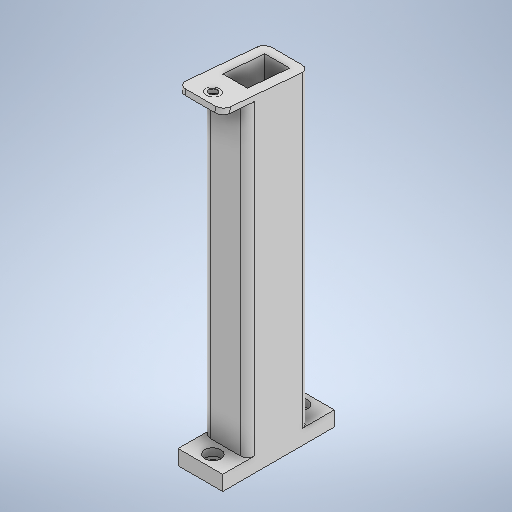
# Autodesk Inventor part: Path Holder
Saved by Autodesk Inventor 2025.4 (Build 294407000, 407)
## iProperties
Created: 2026-04-06
Part Number: Path Holder
Material: Generic
Document SubType Name: Modeling
Designer: lenovo
Density: 1 g/cm^3
Appearance: Default
Author: lenovo
Autodesk Inventor part; units mm, degrees
ref_plane "YZ Plane" through (0, 0, 0) normal (1, 0, 0) x (0, 1, 0)
ref_plane "XZ Plane" through (0, 0, 0) normal (0, 1, 0) x (-1, 0, 0)
ref_plane "XY Plane" through (0, 0, 0) normal (0, 0, 1) x (1, 0, 0)
sketch "Sketch2" plane through (0, 0, 0) normal (0, 1, 0) x (-1, 0, 0)
  line L0 (5, 8.5) -> (-5, 8.5)
  line L1 (-5, 8.5) -> (-5, -8.5)
  line L2 (-5, -8.5) -> (5, -8.5)
  line L3 (5, -8.5) -> (5, 8.5)
  line L4 (5, 8.5) -> (-5, -8.5) construction
  line L5 (-5, 8.5) -> (5, -8.5) construction
  line L6 (9, 12.5) -> (-9, 12.5)
  line L7 (-9, 12.5) -> (-9, -12.5)
  line L8 (-9, -12.5) -> (9, -12.5)
  line L9 (9, -12.5) -> (9, 12.5)
  point P0 (0, 0)
  dimension "d0" = 17
  dimension "d1" = 10
  dimension "d2" = 4
  constraints: 20 end point, 4 parallel, 2 midpoint, 2 perpendicular, 1 horizontal, 3 other
  measures "d0" distance of L2.end L0.start
  measures "d1" distance of L1.end L2.end
  measures "d2" distance between parallel lines of L3 L9
extrude "Extrusion1" add sketch "Sketch2" along normal blind 130
sketch "Sketch3" plane through (9, 0, -12.5) normal (0, 0, -1) x (-1, 0, 0)
  line L0 (0, 0) -> (0, 130) projected
  line L1 (18, 0) -> (18, 130) projected
  line L2 (0, 0) -> (18, 0)
  line L3 (18, 0) -> (18, 6)
  line L4 (18, 6) -> (0, 6)
  line L5 (0, 6) -> (0, 0)
  point P0 (9, 0)
  point P1 (0, 6)
  dimension "d5" = 6
  constraints: 8 end point, 2 parallel, 1 horizontal, 1 perpendicular, 1 point on line
  measures "d5" distance between parallel lines of L2 L4
extrude "Extrusion2" add sketch "Sketch3" along normal blind 10
sketch "Sketch4" plane through (-9, 6, -12.5) normal (0, 1, 0) x (1, 0, 0)
  circle A0 centre (9, 5) radius 3.25
  circle A1 centre (9, 5) radius 1.7
  line L0 (0, 0) -> (0, 10) projected
  line L1 (0, 10) -> (18, 10) projected
  point P0 (9, -12.5)
  point P1 (0, 5)
  point P2 (9, 10)
  dimension "d8" = 6.5
  dimension "d9" = 3.4
  constraints: 2 centre point, 2 midpoint, 1 coincident, 1 horizontal alignment, 1 vertical alignment
  measures "d8" diameter of A0
  measures "d9" diameter of A1
extrude "Extrusion3" cut sketch "Sketch4" against normal blind 10 contours A1
extrude "Extrusion4" cut sketch "Sketch4" against normal blind 3
sketch "Sketch5" plane through (9, 0, 12.5) normal (1, 0, 0) x (0, 0, -1)
  line L0 (0, 0) -> (0, 130) projected
  line L1 (0, 130) -> (0, 132.1872)
  line L2 (25, 130) -> (0, 130) projected
  line L3 (0, 132.1872) -> (25, 130)
  line L4 (0, 132.1872) -> (-9.9619, 133.0588)
  line L5 (-9.9619, 133.0588) -> (-10.1519, 130.8882)
  line L6 (-10.1519, 130.8882) -> (0, 130)
  line L7 (25, 6) -> (25, 130) projected
  point P0 (12.5, 0)
  dimension "d14" = 5
  dimension "d18" = 10
  constraints: 10 end point, 2 perpendicular, 1 parallel, 1 vertical
  measures "d14" angle of L2 L3
  measures "d18" distance of L1.end L4.end
extrude "Extrusion5" add sketch "Sketch5" against normal up to surface (18 mm away)
extrude "Extrusion6" cut sketch "Sketch2" along normal through all contours L3 L2 L1 L0
sketch "Sketch6" plane through (-9, 130, 12.5) normal (0, -0.9961947, 0.0871557) x (1, 0, 0)
  circle A0 centre (9, 5.0953) radius 2.75
  circle A1 centre (9, 5.0953) radius 1.7
  line L0 (0, 10.1906) -> (0, 0) projected
  line L1 (18, 10.1906) -> (0, 10.1906) projected
  point P0 (9, -23.7827)
  point P1 (0, 5.0953)
  point P2 (9, 10.1906)
  dimension "d23" = 5.5
  dimension "d24" = 3.4
  constraints: 2 centre point, 2 midpoint, 1 coincident, 1 horizontal alignment, 1 vertical alignment
  measures "d23" diameter of A0
  measures "d24" diameter of A1
extrude "Extrusion7" cut sketch "Sketch6" against normal blind 10 contours A1
extrude "Extrusion8" cut sketch "Sketch6" against normal blind 2
mirror "Mirror1" about plane through (0, 0, 0) normal (0, 0, 1) of "Extrusion2", "Extrusion3", "Extrusion4"
fillet "Fillet1" radius 3 6 edges at (9, 68, -12.5) (-9, 68, -12.5) (9, 68, 12.5) (-9, 68, 12.5) (9, 131.9735, 22.5569) (-9, 131.9735, 22.5569)
body "Solid1"
